Autodesk Inventor part; units mm, degrees
(part 3 of 3)
  line L224 (2, 5) -> (2, 102.95) projected
  arc A151 (2, 5) -> (5, 2) centre (5, 5) ccw projected
  point P0 (0, 0)
  constraints: 1 horizontal alignment, 1 vertical alignment, 28 other
hole "Hole1" at (5, 102.95, 10) at (63.58, 102.95, 10) at (63.58, 5, 10) at (5, 5, 10) direction (0, 0, -1) diameter 3.4036 end through all clearance for "Flat Head Machine Screw" size "M3" standard "Ansi Metric M Profile"
equation "\"d17\" = d16"
body "Solid1"
